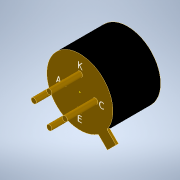
# Autodesk Inventor part: Sensor
Saved by Autodesk Inventor 2022 (Build 260153000, 153)
## iProperties
Created: 2021-10-29
Part Number: Sensor
Material: Generic
Document SubType Name: Modeling
Designer: alber
Density: 1 g/cm^3
Appearance: Default
Author: alber
Autodesk Inventor part; units mm, degrees
ref_plane "YZ Plane" through (0, 0, 0) normal (1, 0, 0) x (0, 1, 0)
ref_plane "XZ Plane" through (0, 0, 0) normal (0, 1, 0) x (-1, 0, 0)
ref_plane "XY Plane" through (0, 0, 0) normal (0, 0, 1) x (1, 0, 0)
sketch "Sketch1" plane through (0, 0, 0) normal (0, 0, 1) x (1, 0, 0)
  circle A0 centre (0, 0) radius 2.7
  dimension "d0" = 5.4
  constraints: 1 centre point, 1 coincident
  measures "d0" diameter of A0
extrude "Extrusion1" add sketch "Sketch1" along normal blind 3.7
sketch "Sketch2" plane through (0, 0, 3.7) normal (0, 0, 1) x (1, 0, 0)
  circle A0 centre (0, 0) radius 1.27
  circle A1 centre (1.27, 0) radius 0.215
  circle A2 centre (0, 1.27) radius 0.215
  circle A3 centre (-1.27, 0) radius 0.215
  circle A4 centre (0, -1.27) radius 0.215
  dimension "d3" = 2.54
  dimension "d4" = 0.43
  dimension "d7" = 360
  constraints: 4 centre point, 1 coincident, 1 horizontal alignment, 11 other
  measures "d4" diameter of A1
extrude "Extrusion2" add sketch "Sketch2" along normal blind 12.7 contours A0 A1 | A0 A1 | A2 A0 | A0 A2 | A4 A0 | A0 A4 | A3 A0 | A0 A3
sketch "Sketch3" plane through (0, 0, 3.7) normal (0, 0, 1) x (1, 0, 0)
  line L0 (2.9561, -2.2765) -> (2.249, -2.9836)
  line L1 (2.249, -2.9836) -> (1.4633, -2.1979)
  line L2 (1.4633, -2.1979) -> (2.1704, -1.4908)
  line L3 (2.1704, -1.4908) -> (2.9561, -2.2765)
  circle A0 centre (0, 0) radius 2.7 projected
  point P0 (2.2185, -1.5389)
  point P1 (1.5062, -2.2408)
  dimension "d11" = 1
  dimension "d12" = 6.4
  constraints: 8 end point, 2 parallel, 1 perpendicular
  measures "d11" distance of L0.start L0.end
extrude "Extrusion3" add sketch "Sketch3" along normal blind 0.2
sketch "Sketch4" plane through (0, 0, 3.9) normal (0, 0, 1) x (1, 0, 0)
  line L0 (-0.2098, -1.6461) -> (0.1759, -1.6461) construction
  line L1 (0.1759, -1.6461) -> (0.1759, -2.1461) construction
  line L2 (0.1759, -2.1461) -> (-0.2098, -2.1461) construction
  line L3 (-0.2098, -2.1461) -> (-0.2098, -1.6461) construction
  line L4 (1.5616, 0.2129) -> (1.9473, 0.2129) construction
  line L5 (1.9473, 0.2129) -> (1.9473, -0.2871) construction
  line L6 (1.9473, -0.2871) -> (1.5616, -0.2871) construction
  line L7 (1.5616, -0.2871) -> (1.5616, 0.2129) construction
  line L8 (-1.9384, 0.2505) -> (-1.5527, 0.2505) construction
  line L9 (-1.5527, 0.2505) -> (-1.5527, -0.2495) construction
  line L10 (-1.5527, -0.2495) -> (-1.9384, -0.2495) construction
  line L11 (-1.9384, -0.2495) -> (-1.9384, 0.2505) construction
  line L12 (-0.1933, 2.1269) -> (0.1924, 2.1269) construction
  line L13 (0.1924, 2.1269) -> (0.1924, 1.6269) construction
  line L14 (0.1924, 1.6269) -> (-0.1933, 1.6269) construction
  line L15 (-0.1933, 1.6269) -> (-0.1933, 2.1269) construction
  point P0 (0, 0)
  constraints: 8 other
move faces "Move1" translate (0, 0, -10) faces at (-0.0635, 1.2367, 16.4) (1.2786, 0.0711, 16.4) (-0.0635, -1.3033, 16.4) (-1.2446, 0.067, 16.4)
body "Solid1"
